Axe 5 v2 (Autodesk Fusion 360 design; units mm, degrees)
Autodesk Fusion 360 part; units mm, degrees
note: some values were not read from the file. Chosen so that the rebuilt part matches the saved one: which face or edge a step refers to. Set by a fixed rule: which sketch regions a step uses.
sketch "Sketch1" plane through (0, 0, 0) normal (0, 0, 1) x (1, 0, 0)
  line L0 (0, 0) -> (0, 16) construction
  line L1 (4.75, 0) -> (-4.75, 0) construction
  line L2 (-4.75, 0) -> (-2.5681, 13.8059)
  line L3 (4.75, 0) -> (2.5681, 13.8059)
  arc A0 (2.5681, 13.8059) -> (-2.5681, 13.8059) centre (0, 13.4) ccw
  line L4 (2.375, 4.1136) -> (-10.6722, 9.127)
  arc A1 (-10.6722, 9.127) -> (-13.2403, 4.6789) centre (-11.6047, 6.7) ccw
  line L5 (-2.375, -4.1136) -> (-13.2403, 4.6789)
  line L6 (-2.375, 4.1136) -> (-13.2403, -4.6789)
  arc A2 (-13.2403, -4.6789) -> (-10.6722, -9.127) centre (-11.6047, -6.7) ccw
  line L7 (2.375, -4.1136) -> (-10.6722, -9.127)
  line L8 (-4.75, 0) -> (-2.5681, -13.8059)
  arc A3 (-2.5681, -13.8059) -> (2.5681, -13.8059) centre (0, -13.4) ccw
  line L9 (4.75, 0) -> (2.5681, -13.8059)
  line L10 (-2.375, -4.1136) -> (10.6722, -9.127)
  arc A4 (10.6722, -9.127) -> (13.2403, -4.6789) centre (11.6047, -6.7) ccw
  line L11 (2.375, 4.1136) -> (13.2403, -4.6789)
  line L12 (2.375, -4.1136) -> (13.2403, 4.6789)
  arc A5 (13.2403, 4.6789) -> (10.6722, 9.127) centre (11.6047, 6.7) ccw
  line L13 (-2.375, 4.1136) -> (10.6722, 9.127)
  circle A6 centre (0, 0) radius 2.1
  circle A7 centre (0, 0) radius 10
  line L14 (-3.4067, 8.5) -> (3.4067, 8.5)
  line L15 (-9.0645, 1.2997) -> (-5.6579, 7.2003)
  line L16 (-5.6579, -7.2003) -> (-9.0645, -1.2997)
  line L17 (3.4067, -8.5) -> (-3.4067, -8.5)
  line L18 (9.0645, -1.2997) -> (5.6579, -7.2003)
  line L19 (5.6579, 7.2003) -> (9.0645, 1.2997)
  dimension "d1" = 16
  dimension "d2" = 5.2
  dimension "d3" = 9.5
  dimension "d5" = 360
  dimension "d6" = 4.2
  dimension "d7" = 20
  dimension "d18" = 8.5
  constraint coincident L0.start A6.centre
  constraint vertical L0
  constraint coincident L0 A0.centre
  constraint coincident L0.end A0
  constraint perpendicular L0 L1
  constraint coincident L0.start L1
  constraint midpoint L0.start L1
  constraint tangent L2 A0
  constraint tangent L3 A0
  constraint coincident L2 L14.start
  constraint coincident L3 L14.end
  constraint perpendicular L0 L14
  measures "d1" distance of L0.start L0.end
  measures "d2" diameter of A0
  measures "d3" distance of L1.start L1.end
  measures "d6" diameter of A6
  measures "d7" diameter of A7
  measures "d18" distance of L0.start L14
extrude "Extrude1" add sketch "Sketch1" along normal blind 3 contours L2 L4 A7 | L5 L6 A7 | L7 L8 A7 | L2 L3 A7 L14 | L4 L5 A7 L15 | L6 L7 A7 L16 | L8 L9 A7 L17 | L3 L13 A7 | L9 L10 A7 | L12 L13 A7 L19 | L10 L11 A7 L18 | L11 L12 A7
extrude "Extrude3" add sketch "Sketch1" against normal blind 5 contours L2 L5 L6 L8 | L2 L3 L4 L5 L6 L7 L8 L9 L10 L11 L12 L13 | L2 L4 L5 L6 L15 | L2 L4 L6 L13 | L5 L6 L7 L8 L16 | L5 L7 L8 L10 | L2 L4 A7 | L2 L3 L4 L13 L14 | L5 L6 A7 | L7 L8 A7 | L7 L8 L9 L10 L17 | L2 L3 A7 L14 | L3 L4 L11 L13 | L4 L5 A7 L15 | L6 L7 A7 L16 | L7 L9 L10 L12 | L8 L9 A7 L17 | L3 L13 A7 | L3 L11 L12 L13 L19 | L9 L10 A7 | L9 L10 L11 L12 L18 | L3 L9 L11 L12 | L12 L13 A7 L19 | L10 L11 A7 L18 | L11 L12 A7
sketch "Sketch2" plane through (0, 0, 0) normal (0, 0, 1) x (-1, 0, 0)
  circle A0 centre (0, 0) radius 2.1
  line L0 (-4.1569, 0) -> (-2.0785, -3.6)
  line L1 (-2.0785, -3.6) -> (2.0785, -3.6)
  line L2 (2.0785, -3.6) -> (4.1569, 0)
  line L3 (4.1569, 0) -> (2.0785, 3.6)
  line L4 (2.0785, 3.6) -> (-2.0785, 3.6)
  line L5 (-2.0785, 3.6) -> (-4.1569, 0)
  line L6 (4.1569, 0) -> (-4.1569, 0) construction
  line L7 (-9.0645, 1.2997) -> (-7.4584, 0)
  line L8 (-7.4584, 0) -> (-9.0645, -1.2997)
  line L9 (-5.6579, -7.2003) -> (-3.7292, -6.4592)
  line L10 (-3.7292, -6.4592) -> (-3.4067, -8.5)
  line L11 (3.4067, -8.5) -> (3.7292, -6.4592)
  line L12 (3.7292, -6.4592) -> (5.6579, -7.2003)
  line L13 (9.0645, -1.2997) -> (7.4584, 0)
  line L14 (7.4584, 0) -> (9.0645, 1.2997)
  line L15 (5.6579, 7.2003) -> (3.7292, 6.4592)
  line L16 (3.7292, 6.4592) -> (3.4067, 8.5)
  line L17 (-3.4067, 8.5) -> (-3.7292, 6.4592)
  line L18 (-3.7292, 6.4592) -> (-5.6579, 7.2003)
  line L19 (-3.4067, -8.5) -> (3.4067, -8.5)
  line L20 (5.6579, -7.2003) -> (9.0645, -1.2997)
  line L21 (9.0645, 1.2997) -> (5.6579, 7.2003)
  line L22 (3.4067, 8.5) -> (-3.4067, 8.5)
  line L23 (-5.6579, 7.2003) -> (-9.0645, 1.2997)
  line L24 (-9.0645, -1.2997) -> (-5.6579, -7.2003)
  dimension "d17" = 7.2
  constraint coincident A0.centre origin
  constraint horizontal L6
  measures "d17" distance of L0 L3
extrude "Extrude4" cut sketch "Sketch2" against normal blind 3.5 contours L0 L1 L2 L3 L4 L5
named bodies: "Axe 5"
